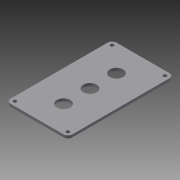
# Autodesk Inventor part: frontplatte
Saved by Autodesk Inventor 2013 (Build 170138000, 138)
## iProperties
Created: 2013-01-11
Part Number: frontplatte
Material: Generic
Document SubType Name: Modeling
Designer: md
Density: 1 g/cm^3
Author: md
Autodesk Inventor part; units mm, degrees
ref_plane "YZ Plane" through (0, 0, 0) normal (1, 0, 0) x (0, 1, 0)
ref_plane "XZ Plane" through (0, 0, 0) normal (0, 1, 0) x (-1, 0, 0)
ref_plane "XY Plane" through (0, 0, 0) normal (0, 0, 1) x (1, 0, 0)
sketch "Sketch1" plane through (0, 0, 0) normal (0, 0, 1) x (1, 0, 0)
  line L0 (30, -60) -> (-30, -60)
  line L1 (-35, -55) -> (-35, 55)
  line L2 (-30, 60) -> (30, 60)
  line L3 (35, 55) -> (35, -55)
  line L4 (-30, -55) -> (30, -55) construction
  line L5 (30, -55) -> (30, 55) construction
  line L6 (30, 55) -> (-30, 55) construction
  line L7 (-30, 55) -> (-30, -55) construction
  line L8 (-30, -55) -> (30, 55) construction
  line L9 (30, -55) -> (-30, 55) construction
  circle A0 centre (-30, 55) radius 2
  circle A1 centre (30, 55) radius 2
  circle A2 centre (30, -55) radius 2
  circle A3 centre (-30, -55) radius 2
  arc A4 (30, -60) -> (35, -55) centre (30, -55) ccw
  arc A5 (-30, 60) -> (-35, 55) centre (-30, 55) ccw
  arc A6 (35, 55) -> (30, 60) centre (30, 55) ccw
  arc A7 (-35, -55) -> (-30, -60) centre (-30, -55) ccw
  circle A8 centre (0, 0) radius 7.55
  circle A9 centre (0, 30) radius 7.55
  circle A10 centre (0, -30) radius 7.55
  dimension "d3" = 5
  dimension "d4" = 5
  dimension "d5" = 4
  dimension "d16" = 60
  dimension "d17" = 120
  dimension "d20" = 15.1
  dimension "d22" = 30
  dimension "d23" = 30
  dimension "d24" = 35
  constraints: 20 end point, 11 centre point, 9 coincident, 8 point on circle, 6 tangent, 5 equal radius, 4 parallel, 2 horizontal, 2 midpoint, 2 perpendicular, 1 vertical alignment
  measures "d3" distance between parallel lines of L6 L2
  measures "d4" distance between parallel lines of L1 L7
  measures "d5" diameter of A1
  measures "d16" distance of L5.end L6.end
  measures "d17" distance between parallel lines of L0 L2
  measures "d20" diameter of A8
  measures "d22" distance of point (0, 0) A9.centre
  measures "d23" distance of point (0, 0) A10.centre
  measures "d24" distance from line of A9.centre L3
extrude "Extrusion2" add sketch "Sketch1" along normal blind 3
equation "\"d3\" = Freistellung_Eckbohrungen"
equation "\"d4\" = d3"
equation "\"d5\" = Durchmesser_Bohrung"
equation "\"d17\" = Hoehe"
equation "\"d20\" = Taster_Durchmesser + epsilon"
equation "\"d22\" = 0.25 * d17"
equation "\"d23\" = d22"
equation "\"d25\" = Plattenstaerke"
equation "\"Plattenstaerke\" = 3"
equation "\"Eckrundung\" = 4"
equation "\"Hoehe\" = 120"
equation "\"Freistellung_Eckbohrungen\" = 5"
equation "\"Durchmesser_Bohrung\" = 4"
equation "\"Taster_Durchmesser\" = 15"
equation "\"epsilon\" = 0.1"
body "Solid2"
